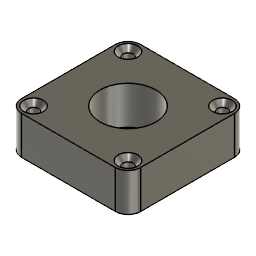
assembly_motor_planetarygear_Wheel (Autodesk Fusion 360 archive; units mm, degrees)
design "MotorHolderFront"
Autodesk Fusion 360 part; units mm, degrees
sketch "Sketch1" plane through (0, 0, 0) normal (0, 0, 1) x (1, 0, 0)
  line L0 (18.75, -18.75) -> (-18.75, -18.75)
  line L1 (-18.75, -18.75) -> (-18.75, 18.75)
  line L2 (-18.75, 18.75) -> (18.75, 18.75)
  line L3 (18.75, 18.75) -> (18.75, -18.75)
  line L4 (18.75, -18.75) -> (-18.75, 18.75) construction
  line L5 (-18.75, -18.75) -> (18.75, 18.75) construction
  line L6 (0, 0) -> (-0.9432, -0.9432)
  line L7 (0, 0) -> (-14.8492, -14.8492)
  circle A0 centre (-14.8492, -14.8492) radius 1.575
  line L8 (0, 5) -> (0, -4)
  line L9 (-5, 0) -> (5, 0)
  circle A1 centre (14.8492, -14.8492) radius 1.575
  circle A2 centre (-14.8492, 14.8492) radius 1.575
  circle A3 centre (14.8492, 14.8492) radius 1.575
  circle A4 centre (0, 0) radius 8.75
  dimension "d3" = 37.5
  dimension "d4" = 37.5
  dimension "d7" = 21
  dimension "d8" = 3.15
  dimension "d13" = 17.5
  constraint horizontal L0
  constraint perpendicular L0 L1
  constraint parallel L0 L2
  constraint parallel L1 L3
  constraint coincident L4 L6.start
  constraint coincident L5 L6.start
  constraint coincident L6.start L7.start
  constraint coincident L5 L6.end
  constraint perpendicular L4 L7
  constraint coincident L7.end A0.centre
  constraint vertical L8
  constraint perpendicular L8 L9
  constraint symmetric A0 L8 A1
  constraint symmetric A0 L9 A2
  constraint symmetric L9 A1 A3
  measures "d3" distance of L1.end L2.end
  measures "d4" distance of L0.end L1.end
  measures "d7" distance of L6.start L7.end
  measures "d8" diameter of A0
  measures "d13" diameter of A4
extrude "Extrude1" add sketch "Sketch1" along normal blind 12
fillet "Fillet1" radius 4 4 edges at (18.75, -18.75, 6) (-18.75, -18.75, 6) (-18.75, 18.75, 6) (18.75, 18.75, 6)
chamfer "Chamfer1" distance 1.5 angle 45 4 edges at (-16.3177, -14.2797, 12) (13.3808, -14.2797, 12) (13.3808, 15.4188, 12) (-16.3177, 15.4188, 12)
sketch "Sketch2" plane through (-18.75, 0, 0) normal (-1, 0, 0) x (0, -1, 0)
  line L0 (-14.75, 12) -> (-14.75, 0)
  line L1 (-14.75, 0) -> (14.75, 0)
  line L2 (14.75, 0) -> (14.75, 12)
  line L3 (14.75, 12) -> (-14.75, 12)
  line L4 (9.5, 6) -> (-9.5, 6)
  line L5 (0, 0) -> (0, 12)
  dimension "d15" = 19
  constraint horizontal L4
  constraint coincident L5.start origin
  constraint midpoint L3 L5.end
  constraint midpoint L4 L5
  measures "d15" distance of L4.start L4.end
hole "Hole1" at (-18.75, 9.5, 6) at (-18.75, -9.5, 6) direction (1, 0, 0) diameter 2.7 depth 12 tip angle 118

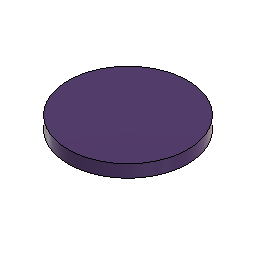
design "protection_front"
Autodesk Fusion 360 part; units mm, degrees
sketch "sketch 547" plane through (0, 0, 8) normal (0, 0, 1) x (-1, 0, 0)
  circle A0 centre (0, 0) radius 14.5
extrude "Extrusion1" add sketch "sketch 547" along normal blind 3
sketch "sketch 560" plane through (0, 0, 11) normal (0, 0, 1) x (-1, 0, 0)
  circle A0 centre (0, 0) radius 14.5
extrude "Extrusion2" add sketch "sketch 560" along normal blind 1
sketch "sketch 572" plane through (0, 0, 12) normal (0, 0, 1) x (-1, 0, 0)
  circle A0 centre (0, 0) radius 17.5
extrude "Extrusion3" add sketch "sketch 572" along normal blind 5
sketch "sketch 584" plane through (0, 0, 8) normal (0, 0, -1) x (1, 0, 0)
  circle A0 centre (8.2087, 4.6771) radius 3
extrude "Extrusion4" cut sketch "sketch 584" against normal blind 3
sketch "sketch 596" plane through (0, 0, 8) normal (0, 0, -1) x (1, 0, 0)
  circle A0 centre (-8.1839, 4.725) radius 2.9
extrude "Extrusion5" cut sketch "sketch 596" against normal blind 3
sketch "sketch 608" plane through (0, 0, 8) normal (0, 0, -1) x (1, 0, 0)
  circle A0 centre (0, -9.45) radius 3.0018
extrude "Extrusion6" cut sketch "sketch 608" against normal blind 3
move_face "Flächen versetzen1" offset -0.1 1 faces at (-5.2875, -4.5804, 10)
move_face "Flächen versetzen2" offset 6.4 1 faces at (-17.4782, -0.8723, 13.6667)

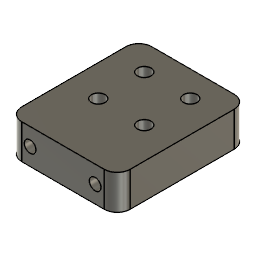
design "MotorHalterHinten"
Autodesk Fusion 360 part; units mm, degrees
sketch "Sketch1" plane through (0, 0, 0) normal (0, 0, 1) x (1, 0, 0)
  line L0 (-12.3588, 26.1654) -> (12.6412, 26.1654)
  line L1 (12.6412, 26.1654) -> (12.6412, -3.8346)
  line L2 (12.6412, -3.8346) -> (-12.3588, -3.8346)
  line L3 (-12.3588, -3.8346) -> (-12.3588, 26.1654)
  line L4 (5.4445, 9.6121) -> (-5.1621, 20.2187)
  line L5 (0.1412, -3.8346) -> (0.1412, 14.9154)
  line L6 (-5.1621, 9.6121) -> (5.4445, 20.2187)
  circle A0 centre (5.4445, 20.2187) radius 1.575
  circle A1 centre (-5.1621, 20.2187) radius 1.575
  circle A2 centre (-5.1621, 9.6121) radius 1.575
  circle A3 centre (5.4445, 9.6121) radius 1.575
  circle A4 centre (0.1412, 14.9154) radius 5.625
  dimension "d1" = 25
  dimension "d2" = 30
  dimension "d10" = 15
  dimension "d11" = 18.75
  dimension "d12" = 15
  dimension "d13" = 135
  dimension "d15" = 3.15
  dimension "d16" = 3.15
  dimension "d17" = 3.15
  dimension "d18" = 3.15
  dimension "d19" = 11.25
  constraint horizontal L0
  constraint vertical L1
  constraint horizontal L2
  constraint vertical L3
  constraint midpoint L2 L5.start
  constraint perpendicular L2 L5
  constraint midpoint L4 L5.end
  constraint midpoint L5.end L6
  constraint perpendicular L4 L6
  constraint coincident L6.end A0.centre
  constraint coincident L4.end A1.centre
  constraint coincident L6.start A2.centre
  constraint coincident L4.start A3.centre
  constraint coincident L5.end A4.centre
  measures "d1" distance of L0.start L0.end
  measures "d2" distance of L0.start L2.end
  measures "d10" distance of L4.start L4.end
  measures "d11" distance of L5.start L5.end
  measures "d12" distance of L6.start L6.end
  measures "d13" angle of L5 L6
  measures "d15" diameter of A0
  measures "d16" diameter of A1
  measures "d17" diameter of A2
  measures "d18" diameter of A3
  measures "d19" diameter of A4
extrude "Extrude1" add sketch "Sketch1" along normal blind 8 contours L0 L1 L2 L3 | L4 L5 A4 | L4 L6 A4 | L4 L6 A4 | L5 L6 A4 | L4 L6 A4
fillet "Fillet1" radius 3 4 edges at (12.6412, 26.1654, 4) (-12.3588, 26.1654, 4) (12.6412, -3.8346, 4) (-12.3588, -3.8346, 4)
extrude "Extrude2" cut sketch "Sketch1" along normal blind 4 contours L4 L5 A4 | L4 L6 A4 | L4 L6 A4 | L5 L6 A4 | L4 L6 A4
sketch "Sketch3" plane through (0, -3.8346, 0) normal (0, -1, 0) x (1, 0, 0)
  line L0 (-9.3588, 8) -> (-9.3588, 0)
  line L1 (-9.3588, 0) -> (9.6412, 0)
  line L2 (9.6412, 0) -> (9.6412, 8)
  line L3 (9.6412, 8) -> (-9.3588, 8)
  line L4 (7.5706, 4) -> (-7.4294, 4)
  line L5 (0, 0) -> (0.1412, 8)
  dimension "d22" = 15
  constraint parallel L3 L4
  constraint coincident L5.start origin
  constraint midpoint L3 L5.end
  constraint midpoint L4 L5
  measures "d22" distance of L4.start L4.end
hole "Hole1" at (-7.4294, -3.8346, 4) at (7.5706, -3.8346, 4) direction (0, 1, 0) diameter 2.7 depth 10 tip angle 118
